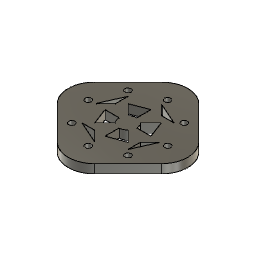
space v4 (Autodesk Fusion 360 design; units mm, degrees)
Autodesk Fusion 360 part; units mm, degrees
note: some values were not read from the file. Set by a fixed rule: which sketch regions a step uses.
sketch "Sketch1" plane through (0, 0, 0) normal (0, 0, 1) x (1, 0, 0)
  line L0 (101.6, 0) -> (101.6, 19.05)
  line L1 (101.6, 19.05) -> (-5.6875, 19.05)
  line L2 (101.6, 0) -> (101.6, -19.05)
  line L3 (101.6, -19.05) -> (-5.6875, -19.05)
  arc A0 (-6.5, 18.9143) -> (-6.5, -18.9143) centre (0, 0) ccw
  arc A1 (-5.6875, 19.05) -> (-6.5, 18.9143) centre (-5.6875, 16.55) ccw
  arc A2 (-6.5, -18.9143) -> (-5.6875, -19.05) centre (-5.6875, -16.55) ccw
  line L4 (0, 0) -> (45, 0) construction
  circle A3 centre (-11.5524, 11.5524) radius 1.5625
  circle A4 centre (11.5524, 11.5524) radius 1.5625
  circle A5 centre (-11.5524, -11.5524) radius 1.5625
  circle A6 centre (11.5524, -11.5524) radius 1.5625
  point P0 (11.5524, -11.5524)
  point P1 (-11.5524, -11.5524)
  point P2 (-11.5524, 11.5524)
  point P3 (11.5524, 11.5524)
  dimension "d1" = 40
  dimension "d2" = 101.6
  dimension "d3" = 19.05
  dimension "d4" = 19.05
  dimension "d5" = 2.5
  dimension "d9" = 3.125
  dimension "d10" = 3.125
  dimension "d11" = 3.125
  dimension "d12" = 3.125
  constraint coincident A0.centre L4.start
  constraint perpendicular L0 L1
  constraint perpendicular L2 L3
  constraint tangent L1 A1
  constraint tangent A0 A1
  constraint tangent L3 A2
  constraint tangent A0 A2
  constraint equal A1 A2
  constraint horizontal L4
  constraint coincident P2 A3.centre
  constraint coincident P3 A4.centre
  constraint coincident P1 A5.centre
  constraint coincident P0 A6.centre
  measures "d1" diameter of A0
  measures "d2" distance of A0.centre L0.start
  measures "d3" distance of L0.start L0.end
  measures "d4" distance of L0.start L2.end
  measures "d5" radius of A1
  measures "d9" diameter of A3
  measures "d10" diameter of A4
  measures "d11" diameter of A5
  measures "d12" diameter of A6
extrude "Extrude1" add sketch "Sketch1" along normal blind 9.525 makes body 1
ref_plane "WorkPlane1" through (47.9563, 0, 4.7625) normal (0, -1, 0) x (1, 0, 0)
pattern_circular "C-Pattern1" count 4 over 360 about axis through (101.6, 0, -2.5717) along (0, 0, 1) of bodies 1 makes body 2 at (101.6, -59.0437, 0) makes body 3 at (160.6437, 0, 0) makes body 4 at (101.6, 59.0437, 0)
combine "Combine1" operation add target body 4 tool bodies 1 2 3
sketch "Sketch2" plane through (0, 0, 9.525) normal (0, 0, 1) x (-1, 0, 0)
  circle A0 centre (-214.7524, -11.5524) radius 1.5625
  circle A1 centre (-191.6476, -11.5524) radius 1.5625
  circle A2 centre (-214.7524, 11.5524) radius 1.5625
  circle A3 centre (-191.6476, 11.5524) radius 1.5625
  line L0 (-120.65, -19.05) -> (-120.65, -107.2875)
  arc A4 (-120.65, -107.2875) -> (-120.5143, -108.1) centre (-118.15, -107.2875) ccw
  arc A5 (-120.5143, -108.1) -> (-82.6857, -108.1) centre (-101.6, -101.6) ccw
  arc A6 (-82.6857, -108.1) -> (-82.55, -107.2875) centre (-85.05, -107.2875) ccw
  line L1 (-82.55, -107.2875) -> (-82.55, -19.05)
  line L2 (-82.55, -19.05) -> (5.6875, -19.05)
  arc A7 (5.6875, -19.05) -> (6.5, -18.9143) centre (5.6875, -16.55) ccw
  arc A8 (6.5, -18.9143) -> (6.5, 18.9143) centre (0, 0) ccw
  arc A9 (6.5, 18.9143) -> (5.6875, 19.05) centre (5.6875, 16.55) ccw
  line L3 (5.6875, 19.05) -> (-82.55, 19.05)
  line L4 (-82.55, 19.05) -> (-82.55, 107.2875)
  arc A10 (-82.55, 107.2875) -> (-82.6857, 108.1) centre (-85.05, 107.2875) ccw
  arc A11 (-82.6857, 108.1) -> (-120.5143, 108.1) centre (-101.6, 101.6) ccw
  arc A12 (-120.5143, 108.1) -> (-120.65, 107.2875) centre (-118.15, 107.2875) ccw
  line L5 (-120.65, 107.2875) -> (-120.65, 19.05)
  line L6 (-120.65, 19.05) -> (-208.8875, 19.05)
  arc A13 (-208.8875, 19.05) -> (-209.7, 18.9143) centre (-208.8875, 16.55) ccw
  arc A14 (-209.7, 18.9143) -> (-209.7, -18.9143) centre (-203.2, 0) ccw
  arc A15 (-209.7, -18.9143) -> (-208.8875, -19.05) centre (-208.8875, -16.55) ccw
  line L7 (-208.8875, -19.05) -> (-120.65, -19.05)
  circle A16 centre (-90.0476, 90.0476) radius 1.5625
  circle A17 centre (-90.0476, 113.1524) radius 1.5625
  circle A18 centre (-113.1524, 90.0476) radius 1.5625
  circle A19 centre (-113.1524, 113.1524) radius 1.5625
  circle A20 centre (-90.0476, -113.1524) radius 1.5625
  circle A21 centre (-90.0476, -90.0476) radius 1.5625
  circle A22 centre (-113.1524, -113.1524) radius 1.5625
  circle A23 centre (-113.1524, -90.0476) radius 1.5625
  circle A24 centre (11.5524, 11.5524) radius 1.5625
  circle A25 centre (-11.5524, 11.5524) radius 1.5625
  circle A26 centre (11.5524, -11.5524) radius 1.5625
  circle A27 centre (-11.5524, -11.5524) radius 1.5625
  line L8 (-52.9071, -19.05) -> (-82.55, -47.7089)
  line L9 (-120.65, -46.4135) -> (-147.0929, -19.05)
  line L10 (-147.0929, 19.05) -> (-120.65, 46.4135)
  line L11 (-82.55, 47.7089) -> (-52.9071, 19.05)
  constraint coincident L2 L8.start
  constraint coincident L1 L8.end
  constraint coincident L0 L9.start
  constraint coincident L7 L9.end
  constraint coincident L6 L10.start
  constraint coincident L5 L10.end
  constraint coincident L4 L11.start
  constraint coincident L3 L11.end
extrude "Extrude2" add sketch "Sketch2" against normal up to surface (9.525 mm away) contours L0 L7 L9 | L1 L2 L8 | L5 L6 L10 | L3 L4 L11 bodies 4
sketch "Sketch3" plane through (0, 0, 0) normal (0, 0, -1) x (1, 0, 0)
  circle A0 centre (191.6476, 11.5524) radius 1.5625
  circle A1 centre (214.7524, 11.5524) radius 1.5625
  circle A2 centre (191.6476, -11.5524) radius 1.5625
  circle A3 centre (214.7524, -11.5524) radius 1.5625
  circle A4 centre (113.1524, -90.0476) radius 1.5625
  circle A5 centre (113.1524, -113.1524) radius 1.5625
  circle A6 centre (90.0476, -90.0476) radius 1.5625
  circle A7 centre (90.0476, -113.1524) radius 1.5625
  circle A8 centre (11.5524, -11.5524) radius 1.5625
  circle A9 centre (-11.5524, -11.5524) radius 1.5625
  circle A10 centre (11.5524, 11.5524) radius 1.5625
  circle A11 centre (-11.5524, 11.5524) radius 1.5625
  line L0 (120.65, 46.4135) -> (120.65, 107.2875)
  arc A12 (120.65, 107.2875) -> (120.5143, 108.1) centre (118.15, 107.2875) ccw
  arc A13 (120.5143, 108.1) -> (82.6857, 108.1) centre (101.6, 101.6) ccw
  arc A14 (82.6857, 108.1) -> (82.55, 107.2875) centre (85.05, 107.2875) ccw
  line L1 (82.55, 107.2875) -> (82.55, 47.7089)
  line L2 (82.55, 47.7089) -> (52.9071, 19.05)
  line L3 (52.9071, 19.05) -> (-5.6875, 19.05)
  arc A15 (-5.6875, 19.05) -> (-6.5, 18.9143) centre (-5.6875, 16.55) ccw
  arc A16 (-6.5, 18.9143) -> (-6.5, -18.9143) centre (0, 0) ccw
  arc A17 (-6.5, -18.9143) -> (-5.6875, -19.05) centre (-5.6875, -16.55) ccw
  line L4 (-5.6875, -19.05) -> (52.9071, -19.05)
  line L5 (52.9071, -19.05) -> (82.55, -47.7089)
  line L6 (82.55, -47.7089) -> (82.55, -107.2875)
  arc A18 (82.55, -107.2875) -> (82.6857, -108.1) centre (85.05, -107.2875) ccw
  arc A19 (82.6857, -108.1) -> (120.5143, -108.1) centre (101.6, -101.6) ccw
  arc A20 (120.5143, -108.1) -> (120.65, -107.2875) centre (118.15, -107.2875) ccw
  line L7 (120.65, -107.2875) -> (120.65, -46.4135)
  line L8 (120.65, -46.4135) -> (147.0929, -19.05)
  line L9 (147.0929, -19.05) -> (208.8875, -19.05)
  arc A21 (208.8875, -19.05) -> (209.7, -18.9143) centre (208.8875, -16.55) ccw
  arc A22 (209.7, -18.9143) -> (209.7, 18.9143) centre (203.2, 0) ccw
  arc A23 (209.7, 18.9143) -> (208.8875, 19.05) centre (208.8875, 16.55) ccw
  line L10 (208.8875, 19.05) -> (147.0929, 19.05)
  line L11 (147.0929, 19.05) -> (120.65, 46.4135)
  circle A24 centre (90.0476, 90.0476) radius 1.5625
  circle A25 centre (90.0476, 113.1524) radius 1.5625
  circle A26 centre (113.1524, 90.0476) radius 1.5625
  circle A27 centre (113.1524, 113.1524) radius 1.5625
  circle A28 centre (77.5495, 0.0251) radius 1.727
  circle A29 centre (100, 22.4505) radius 1.727
  circle A30 centre (122.4505, 0) radius 1.727
  circle A31 centre (99.9787, -22.4505) radius 1.727
  circle A32 centre (73.0825, 26.964) radius 1.727
  circle A33 centre (126.964, 26.9175) radius 1.727
  circle A34 centre (126.9175, -26.964) radius 1.727
  circle A35 centre (73.036, -26.9175) radius 1.727
  dimension "d21" = 3.454
  dimension "d22" = 3.454
  dimension "d23" = 3.454
  dimension "d24" = 3.454
  dimension "d26" = 3.454
  dimension "d27" = 3.454
  dimension "d28" = 3.454
  dimension "d29" = 3.454
  measures "d21" diameter of A28
  measures "d22" diameter of A29
  measures "d23" diameter of A30
  measures "d24" diameter of A31
  measures "d26" diameter of A32
  measures "d27" diameter of A33
  measures "d28" diameter of A34
  measures "d29" diameter of A35
extrude "Extrude3" cut sketch "Sketch3" against normal blind 10 contours A28 | A29 | A30 | A31 | A32 | A33 | A34 | A35 bodies 4
sketch "Sketch4" plane through (0, 0, 9.525) normal (0, 0, 1) x (-1, 0, 0)
  circle A0 centre (-122.4505, 0) radius 1.727
  circle A1 centre (-77.5495, 0.0251) radius 1.727
  circle A2 centre (-73.036, -26.9175) radius 1.727
  circle A3 centre (-100, 22.4505) radius 1.727
  circle A4 centre (-126.9175, -26.964) radius 1.727
  circle A5 centre (-73.0825, 26.964) radius 1.727
  circle A6 centre (-99.9787, -22.4505) radius 1.727
  circle A7 centre (-126.964, 26.9175) radius 1.727
  circle A8 centre (-214.7524, -11.5524) radius 1.5625
  circle A9 centre (-191.6476, -11.5524) radius 1.5625
  circle A10 centre (-214.7524, 11.5524) radius 1.5625
  circle A11 centre (-191.6476, 11.5524) radius 1.5625
  line L0 (-120.65, -46.4135) -> (-120.65, -107.2875)
  arc A12 (-120.65, -107.2875) -> (-120.5143, -108.1) centre (-118.15, -107.2875) ccw
  arc A13 (-120.5143, -108.1) -> (-82.6857, -108.1) centre (-101.6, -101.6) ccw
  arc A14 (-82.6857, -108.1) -> (-82.55, -107.2875) centre (-85.05, -107.2875) ccw
  line L1 (-82.55, -107.2875) -> (-82.55, -47.7089)
  line L2 (-82.55, -47.7089) -> (-52.9071, -19.05)
  line L3 (-52.9071, -19.05) -> (5.6875, -19.05)
  arc A15 (5.6875, -19.05) -> (6.5, -18.9143) centre (5.6875, -16.55) ccw
  arc A16 (6.5, -18.9143) -> (6.5, 18.9143) centre (0, 0) ccw
  arc A17 (6.5, 18.9143) -> (5.6875, 19.05) centre (5.6875, 16.55) ccw
  line L4 (5.6875, 19.05) -> (-52.9071, 19.05)
  line L5 (-52.9071, 19.05) -> (-82.55, 47.7089)
  line L6 (-82.55, 47.7089) -> (-82.55, 107.2875)
  arc A18 (-82.55, 107.2875) -> (-82.6857, 108.1) centre (-85.05, 107.2875) ccw
  arc A19 (-82.6857, 108.1) -> (-120.5143, 108.1) centre (-101.6, 101.6) ccw
  arc A20 (-120.5143, 108.1) -> (-120.65, 107.2875) centre (-118.15, 107.2875) ccw
  line L7 (-120.65, 107.2875) -> (-120.65, 46.4135)
  line L8 (-120.65, 46.4135) -> (-147.0929, 19.05)
  line L9 (-147.0929, 19.05) -> (-208.8875, 19.05)
  arc A21 (-208.8875, 19.05) -> (-209.7, 18.9143) centre (-208.8875, 16.55) ccw
  arc A22 (-209.7, 18.9143) -> (-209.7, -18.9143) centre (-203.2, 0) ccw
  arc A23 (-209.7, -18.9143) -> (-208.8875, -19.05) centre (-208.8875, -16.55) ccw
  line L10 (-208.8875, -19.05) -> (-147.0929, -19.05)
  line L11 (-147.0929, -19.05) -> (-120.65, -46.4135)
  circle A24 centre (-90.0476, 90.0476) radius 1.5625
  circle A25 centre (-90.0476, 113.1524) radius 1.5625
  circle A26 centre (-113.1524, 90.0476) radius 1.5625
  circle A27 centre (-113.1524, 113.1524) radius 1.5625
  circle A28 centre (-90.0476, -113.1524) radius 1.5625
  circle A29 centre (-90.0476, -90.0476) radius 1.5625
  circle A30 centre (-113.1524, -113.1524) radius 1.5625
  circle A31 centre (-113.1524, -90.0476) radius 1.5625
  circle A32 centre (11.5524, 11.5524) radius 1.5625
  circle A33 centre (-11.5524, 11.5524) radius 1.5625
  circle A34 centre (11.5524, -11.5524) radius 1.5625
  circle A35 centre (-11.5524, -11.5524) radius 1.5625
  line L12 (-72.5, 27.5) -> (-127.5, -27.5) construction
  line L13 (-127.5, 27.5) -> (-72.5, -27.5) construction
  line L14 (-72.5, 0) -> (-100, 27.5)
  line L15 (-100, 27.5) -> (-127.5, 0)
  line L16 (-127.5, 0) -> (-100, -27.5)
  line L17 (-72.5, 0) -> (-100, -27.5)
  line L18 (-127.5, -27.5) -> (-125.2758, -27.5)
  line L19 (-74.6618, -27.5) -> (-72.5, -27.5)
  line L20 (-72.5, -27.5) -> (-72.5, -25.2758)
  line L21 (-72.5, 25.3382) -> (-72.5, 27.5)
  line L22 (-127.5, 27.5) -> (-127.5, 25.2758)
  line L23 (-127.5, -25.3382) -> (-127.5, -27.5)
  line L24 (-72.5, 27.5) -> (-74.7242, 27.5)
  line L25 (-125.3382, 27.5) -> (-127.5, 27.5)
  circle A36 centre (-100, 0) radius 141.4214
  point P0 (-100, 0)
  dimension "d32" = 55
  dimension "d33" = 55
  constraint horizontal L24
  constraint perpendicular L22 L24
  constraint parallel L18 L24
  constraint parallel L20 L22
  constraint coincident L12 P0
  constraint coincident L13 P0
  constraint coincident A2 L19.start
  constraint collinear L18 L19
  constraint coincident A2 L20.end
  constraint collinear L20 L21
  constraint coincident L14.start L20
  constraint coincident A4 L18.end
  constraint coincident A4 L23.start
  constraint collinear L22 L23
  constraint coincident A7 L22.end
  constraint coincident A7 L25.start
  constraint collinear L24 L25
  constraint coincident A5 L24.end
  constraint coincident A5 L21.start
  constraint coincident P0 A36.centre
  measures "d32" distance of L12.end L13.end
  measures "d33" distance of L13.start L12.end
extrude "Extrude4" cut sketch "Sketch4" against normal blind 80 contours L0 A12 A13 A14 L1 L2 L3 A15 A16 A17 L4 L5 L6 A18 A19 A20 L7 L8 L9 A21 A22 A23 L10 L11 bodies 4
sketch "Sketch5" plane through (63.75, -63.75, 0) normal (0.707107, -0.707107, 0) x (0.707107, 0.707107, 0)
  line L0 (51.2652, 0) -> (90.1561, 0)
  line L1 (90.1561, 0) -> (90.1561, 9.525)
  line L2 (90.1561, 9.525) -> (51.2652, 9.525)
  line L3 (51.2652, 9.525) -> (51.2652, 0)
  line L4 (51.2652, 4.7625) -> (90.1561, 4.7625)
  constraint midpoint L3 L4.start
  constraint midpoint L1 L4.end
extrude "Extrude5" cut sketch "Sketch5" against normal blind 135 contours L0 L1 L3 L4 bodies 4
fillet "Fillet1" radius 2.5 4 edges at (100, -27.5, 7.1438) (127.5, 0, 7.1438) (100, 27.5, 7.1438) (72.5, 0, 7.1438) on bodies 4
sketch "Sketch6" plane through (0, 0, 9.525) normal (0, 0, 1) x (-1, 0, 0)
  arc A0 (-74.2678, -1.7678) -> (-74.2678, 1.7678) centre (-76.0355, 0) ccw
  line L0 (-74.2678, 1.7678) -> (-98.2322, 25.7322)
  arc A1 (-98.2322, 25.7322) -> (-101.7678, 25.7322) centre (-100, 23.9645) ccw
  line L1 (-101.7678, 25.7322) -> (-125.7322, 1.7678)
  arc A2 (-125.7322, 1.7678) -> (-125.7322, -1.7678) centre (-123.9645, 0) ccw
  line L2 (-125.7322, -1.7678) -> (-101.7678, -25.7322)
  arc A3 (-101.7678, -25.7322) -> (-98.2322, -25.7322) centre (-100, -23.9645) ccw
  line L3 (-98.2322, -25.7322) -> (-74.2678, -1.7678)
  circle A4 centre (-122.4505, 0) radius 1.727
  circle A5 centre (-77.5495, 0.0251) radius 1.727
  circle A6 centre (-100, 22.4505) radius 1.727
  circle A7 centre (-99.9787, -22.4505) radius 1.727
  line L4 (-100, -40) -> (-140, 0)
  line L5 (-140, 0) -> (-100, 40)
  line L6 (-100, 40) -> (-60, 0)
  line L7 (-60, 0) -> (-100, -40)
  constraint perpendicular L4 L5
  constraint perpendicular L5 L6
  constraint perpendicular L4 L7
extrude "Extrude6" add sketch "Sketch6" against normal blind 5 contours L4 L5 L6 L7 bodies 4
sketch "Sketch7" plane through (0, 0, 9.525) normal (0, 0, 1) x (-1, 0, 0)
  line L0 (-60, 0) -> (-100, 40)
  line L1 (-100, 40) -> (-140, 0)
  line L2 (-140, 0) -> (-100, -40)
  line L3 (-100, -40) -> (-60, 0)
  circle A0 centre (-122.4505, 0) radius 1.727
  circle A1 centre (-77.5495, 0.0251) radius 1.727
  circle A2 centre (-100, 22.4505) radius 1.727
  circle A3 centre (-99.9787, -22.4505) radius 1.727
  circle A4 centre (-100, 0) radius 22.5
  line L4 (-100, 0) -> (-120, 20)
  line L5 (-100, 0) -> (-80, -20)
  line L6 (-100, 0) -> (-120, -20)
  line L7 (-100, 0) -> (-80, 20)
  circle A5 centre (-84.0901, -15.9099) radius 1.727
  circle A6 centre (-115.9099, -15.9099) radius 1.727
  circle A7 centre (-115.9099, 15.9099) radius 1.727
  circle A8 centre (-84.0901, 15.9099) radius 1.727
  dimension "d42" = 45
  dimension "d43" = 3.454
  dimension "d44" = 3.454
  dimension "d45" = 3.454
  dimension "d46" = 3.454
  constraint coincident A4.centre L4.start
  constraint midpoint L1 L4.end
  constraint midpoint L3 L5.end
  constraint midpoint L2 L6.end
  constraint midpoint L0 L7.end
  constraint coincident A4 A5.centre
  constraint coincident L5 A5.centre
  constraint coincident A4 A6.centre
  constraint coincident L6 A6.centre
  constraint coincident A4 A7.centre
  constraint coincident L4 A7.centre
  constraint coincident A4 A8.centre
  constraint coincident L7 A8.centre
  measures "d42" diameter of A4
  measures "d43" diameter of A5
  measures "d44" diameter of A6
  measures "d45" diameter of A7
  measures "d46" diameter of A8
extrude "Extrude7" cut sketch "Sketch7" against normal blind 6 contours A4 L7 A8 | A4 L7 A8 | A4 L5 A5 | A4 L5 A5 | A4 L7 A8 | A4 L7 A8 | A4 L5 A5 | A4 L5 A5 | A4 L4 A7 | A4 L4 A7 | A4 L6 A6 | A4 L6 A6 | A4 L4 A7 | A4 L4 A7 | A4 L6 A6 | A4 L6 A6 bodies 4
fillet "Fillet2" radius 15 4 edges at (60, 0, 7.025) (100, -40, 7.025) (140, 0, 7.025) (100, 40, 7.025) on bodies 4
sketch "Sketch8" plane through (0, 0, 9.525) normal (0, 0, 1) x (-1, 0, 0)
  circle A0 centre (-115.9099, -15.9099) radius 1.727
  circle A1 centre (-115.9099, 15.9099) radius 1.727
  circle A2 centre (-84.0901, -15.9099) radius 1.727
  circle A3 centre (-84.0901, 15.9099) radius 1.727
  arc A4 (-110.6066, -29.3934) -> (-89.3934, -29.3934) centre (-100, -18.7868) ccw
  line L0 (-89.3934, -29.3934) -> (-70.6066, -10.6066)
  arc A5 (-70.6066, -10.6066) -> (-70.6066, 10.6066) centre (-81.2132, 0) ccw
  line L1 (-70.6066, 10.6066) -> (-89.3934, 29.3934)
  arc A6 (-89.3934, 29.3934) -> (-110.6066, 29.3934) centre (-100, 18.7868) ccw
  line L2 (-110.6066, 29.3934) -> (-129.3934, 10.6066)
  arc A7 (-129.3934, 10.6066) -> (-129.3934, -10.6066) centre (-118.7868, 0) ccw
  line L3 (-129.3934, -10.6066) -> (-110.6066, -29.3934)
  circle A8 centre (-122.4505, 0) radius 1.727
  circle A9 centre (-77.5495, 0.0251) radius 1.727
  circle A10 centre (-100, 22.4505) radius 1.727
  circle A11 centre (-99.9787, -22.4505) radius 1.727
  circle A12 centre (-100, 0) radius 18.3848
  line L4 (-87, -13) -> (-113, -13)
  line L5 (-113, -13) -> (-113, 13)
  line L6 (-113, 13) -> (-87, 13)
  line L7 (-87, 13) -> (-87, -13)
  line L8 (-87, -13) -> (-88, -12)
  line L9 (-88, -12) -> (-113, 13)
  line L10 (-87, 13) -> (-113, -13)
  line L11 (-81.6152, 0) -> (-118.7868, 0)
  line L12 (-100, -18.7868) -> (-100, 18.7868)
  line L13 (-87, -13) -> (-100, -18.7868)
  line L14 (-100, -18.7868) -> (-113, -13)
  line L15 (-81.2132, 0) -> (-87, -13)
  line L16 (-81.2132, 0) -> (-87, 13)
  line L17 (-100, 18.7868) -> (-87, 13)
  line L18 (-100, 18.7868) -> (-113, 13)
  line L19 (-118.7868, 0) -> (-113, 13)
  line L20 (-118.7868, 0) -> (-113, -13)
  line L21 (-81.2132, 0) -> (-100, -18.7868)
  line L22 (-100, -18.7868) -> (-118.8934, 0.1066)
  line L23 (-118.8934, 0.1066) -> (-100.1066, 18.8934)
  line L24 (-100.1066, 18.8934) -> (-81.2132, 0)
  line L25 (-87, 0) -> (-90.6066, -9.3934)
  line L26 (-100, -13) -> (-90.6066, -9.3934)
  line L27 (-100, -13) -> (-109.4467, -9.3401)
  line L28 (-109.4467, -9.3401) -> (-113, 0)
  line L29 (-113, 0) -> (-109.5, 9.5)
  line L30 (-109.5, 9.5) -> (-100, 13)
  line L31 (-100, 13) -> (-90.6599, 9.4467)
  line L32 (-87, 0) -> (-90.6599, 9.4467)
  circle A13 centre (-100, 0) radius 5
  constraint horizontal L4
  constraint vertical L5
  constraint horizontal L6
  constraint vertical L7
  constraint coincident A12 L5.end
  constraint coincident A12 L4.start
  constraint parallel L8 L9
  constraint perpendicular L9 L10
  constraint coincident A12 L11.start
  constraint coincident A7.centre L11.end
  constraint perpendicular L5 L11
  constraint coincident A4.centre L12.start
  constraint coincident A6.centre L12.end
  constraint coincident A5.centre L15.start
  constraint perpendicular L21 L22
  constraint parallel L21 L23
  constraint parallel L22 L24
  constraint midpoint L7 L25.start
  constraint midpoint L21 L25.end
  constraint midpoint L4 L26.start
  constraint midpoint L22 L27.end
  constraint midpoint L5 L28.end
  constraint midpoint L23 L29.end
  constraint midpoint L6 L30.end
  constraint midpoint L24 L31.end
  constraint concentric A12 A13
extrude "Extrude8" cut sketch "Sketch8" against normal blind 24 contours A12 L7 L15 L21 | L10 L11 L32 A13 | L9 L12 L26 A13 | A12 L6 L17 L24 | L9 L12 L30 A13 | L10 L11 L27 L28 A13 | A12 L4 L14 L22 | A12 L5 L19 L23 bodies 4
extrude "Extrude9" add 1 faces at (115.7282, 4.7249, 4.7625) along direction (0, 0, -1) up to surface (0.2375 mm away) on bodies 4 bodies 4
